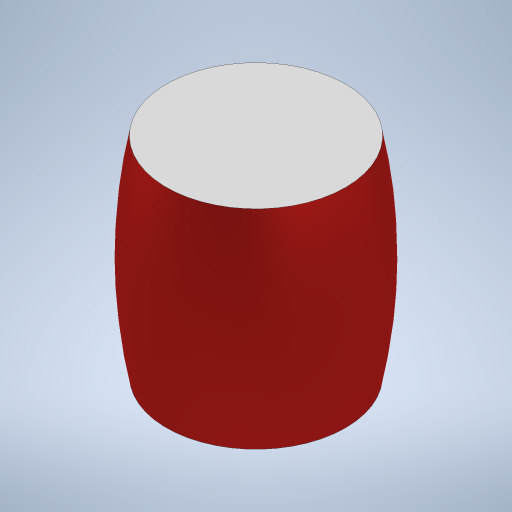
# Autodesk Inventor part: Part1
Saved by Autodesk Inventor 2024 (Build 280153000, 153)
## iProperties
Created: 2024-02-11
Part Number: Part1
Material: Generic
Document SubType Name: Modeling
Designer: HP
Density: 1 g/cm^3
Appearance: Default
Author: HP
Autodesk Inventor part; units mm, degrees
ref_plane "YZ Plane" through (0, 0, 0) normal (1, 0, 0) x (0, 1, 0)
ref_plane "XZ Plane" through (0, 0, 0) normal (0, 1, 0) x (-1, 0, 0)
ref_plane "XY Plane" through (0, 0, 0) normal (0, 0, 1) x (1, 0, 0)
sketch "Sketch1" plane through (0, 0, 0) normal (0, 0, 1) x (1, 0, 0)
  line L0 (0, 0) -> (0, 454.55)
  line L1 (0, 454.55) -> (195.371, 454.55)
  line L2 (0, 454.55) -> (-179.5834, 454.55)
  line L3 (-179.5834, 454.55) -> (-179.5834, -8.5516)
  line L4 (0, -169.0584) -> (195.371, -169.0584)
  line L5 (0, 0) -> (195.371, 0)
  arc A0 (195.371, 0) -> (195.371, 454.55) centre (-924.8054, 227.275) ccw
  dimension "d0" = 1143
  constraints: 12 end point, 2 point on circle, 1 centre point, 1 horizontal, 1 vertical
  measures "d0" radius of A0
revolve "Revolution1" add sketch "Sketch1" angle 360 about axis through (0, 0, 0) along (0, 1, 0)
body "Solid1"
